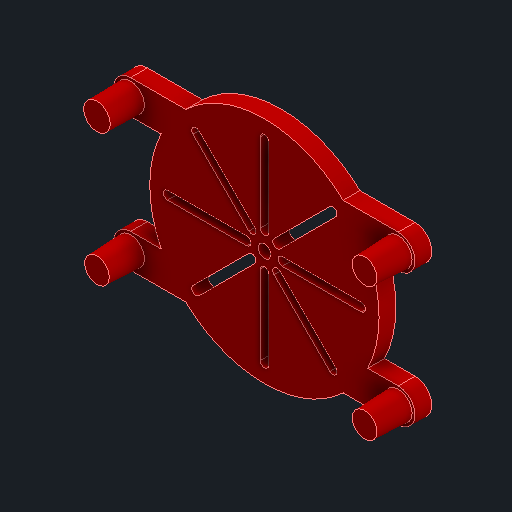
# Autodesk Inventor part: Laser Alignment Tool V2
Saved by Autodesk Inventor 2023.4 (Build 274418000, 418)
## iProperties
Created: 2022-11-15
Part Number: Laser Alignment Tool V2
Material: Generic
Document SubType Name: Modeling
Designer: xSibe
Density: 1 g/cm^3
Appearance: Plastic Dark Red
Author: xSibe
Autodesk Inventor part; units mm, degrees
ref_plane "YZ Plane" through (0, 0, 0) normal (1, 0, 0) x (0, 1, 0)
ref_plane "XZ Plane" through (0, 0, 0) normal (0, 1, 0) x (-1, 0, 0)
ref_plane "XY Plane" through (0, 0, 0) normal (0, 0, 1) x (1, 0, 0)
sketch "Sketch2" plane through (0, 0, 0) normal (0, 0, 1) x (0, 1, 0)
  line L0 (7.7, -24.9) -> (42.1, -24.9) projected
  line L1 (7.7, -24.9) -> (42.1, -24.9) projected
  circle A0 centre (34.8, 19.9) radius 2.0625 projected
  circle A1 centre (15, 19.9) radius 2.0625 projected
  circle A2 centre (15, -19.9) radius 2.0625 projected
  circle A3 centre (34.8, -19.9) radius 2.0625 projected
  line L2 (7.7, 17.05) -> (42.1, 17.05) projected
  line L3 (7.7, -17.05) -> (42.1, -17.05) projected
  line L4 (24.9, 17.05) -> (24.9, -17.05)
  circle A4 centre (24.9, 0) radius 17.05
  circle A5 centre (24.9, 0) radius 0.9375
  line L5 (24.9, 0) -> (36.9562, -12.0562)
  line L6 (24.9, 0) -> (41.95, 0) construction
  line L7 (26.7738, -1.8738) -> (35.0823, -10.1823) construction
  line L8 (26.3319, -2.3158) -> (34.6404, -10.6243)
  line L9 (35.5243, -9.7404) -> (27.2158, -1.4319)
  arc A6 (27.2158, -1.4319) -> (26.3319, -2.3158) centre (26.7738, -1.8738) ccw
  arc A7 (34.6404, -10.6243) -> (35.5243, -9.7404) centre (35.0823, -10.1823) ccw
  line L10 (30.9281, -6.0281) -> (42.6781, -6.0281) construction
  line L11 (34.8, 19.9) -> (34.8, 13.8814) construction
  line L12 (32.3, 19.9) -> (32.3, 13.8814)
  line L13 (37.3, 13.8814) -> (37.3, 19.9)
  arc A8 (37.3, 19.9) -> (32.3, 19.9) centre (34.8, 19.9) ccw
  arc A9 (32.3, 13.8814) -> (37.3, 13.8814) centre (34.8, 13.8814) ccw
  line L14 (15, 19.9) -> (15, 13.8814) construction
  line L15 (12.5, 19.9) -> (12.5, 13.8814)
  line L16 (17.5, 13.8814) -> (17.5, 19.9)
  arc A10 (17.5, 19.9) -> (12.5, 19.9) centre (15, 19.9) ccw
  arc A11 (12.5, 13.8814) -> (17.5, 13.8814) centre (15, 13.8814) ccw
  line L17 (15, -19.9) -> (15, -13.8814) construction
  line L18 (17.5, -19.9) -> (17.5, -13.8814)
  line L19 (12.5, -13.8814) -> (12.5, -19.9)
  arc A12 (12.5, -19.9) -> (17.5, -19.9) centre (15, -19.9) ccw
  arc A13 (17.5, -13.8814) -> (12.5, -13.8814) centre (15, -13.8814) ccw
  line L20 (34.8, -19.9) -> (34.8, -13.8814) construction
  line L21 (37.3, -19.9) -> (37.3, -13.8814)
  line L22 (32.3, -13.8814) -> (32.3, -19.9)
  arc A14 (32.3, -19.9) -> (37.3, -19.9) centre (34.8, -19.9) ccw
  arc A15 (37.3, -13.8814) -> (32.3, -13.8814) centre (34.8, -13.8814) ccw
  line L23 (39.3, 0.625) -> (27.55, 0.625)
  arc A16 (39.3, -0.625) -> (39.3, 0.625) centre (39.3, 0) ccw
  line L24 (27.55, -0.625) -> (39.3, -0.625)
  arc A17 (27.55, 0.625) -> (27.55, -0.625) centre (27.55, 0) ccw
  line L25 (34.6404, 10.6243) -> (26.3319, 2.3158)
  arc A18 (35.5243, 9.7404) -> (34.6404, 10.6243) centre (35.0823, 10.1823) ccw
  line L26 (27.2158, 1.4319) -> (35.5243, 9.7404)
  arc A19 (26.3319, 2.3158) -> (27.2158, 1.4319) centre (26.7738, 1.8738) ccw
  line L27 (24.275, 14.4) -> (24.275, 2.65)
  arc A20 (25.525, 14.4) -> (24.275, 14.4) centre (24.9, 14.4) ccw
  line L28 (25.525, 2.65) -> (25.525, 14.4)
  arc A21 (24.275, 2.65) -> (25.525, 2.65) centre (24.9, 2.65) ccw
  line L29 (14.2757, 9.7404) -> (22.5842, 1.4319)
  arc A22 (15.1596, 10.6243) -> (14.2757, 9.7404) centre (14.7177, 10.1823) ccw
  line L30 (23.4681, 2.3158) -> (15.1596, 10.6243)
  arc A23 (22.5842, 1.4319) -> (23.4681, 2.3158) centre (23.0262, 1.8738) ccw
  line L31 (10.5, -0.625) -> (22.25, -0.625)
  arc A24 (10.5, 0.625) -> (10.5, -0.625) centre (10.5, 0) ccw
  line L32 (22.25, 0.625) -> (10.5, 0.625)
  arc A25 (22.25, -0.625) -> (22.25, 0.625) centre (22.25, 0) ccw
  line L33 (15.1596, -10.6243) -> (23.4681, -2.3158)
  arc A26 (14.2757, -9.7404) -> (15.1596, -10.6243) centre (14.7177, -10.1823) ccw
  line L34 (22.5842, -1.4319) -> (14.2757, -9.7404)
  arc A27 (23.4681, -2.3158) -> (22.5842, -1.4319) centre (23.0262, -1.8738) ccw
  line L35 (25.525, -14.4) -> (25.525, -2.65)
  arc A28 (24.275, -14.4) -> (25.525, -14.4) centre (24.9, -14.4) ccw
  line L36 (24.275, -2.65) -> (24.275, -14.4)
  arc A29 (25.525, -2.65) -> (24.275, -2.65) centre (24.9, -2.65) ccw
  line L37 (37.3, 13.8814) -> (37.3, -13.8814)
  line L38 (12.5, -13.8814) -> (12.5, 13.8814)
  point P0 (0, 0)
  point P1 (34.8, 16.8907)
  point P2 (15, 16.8907)
  point P3 (15, -16.8907)
  point P4 (34.8, -16.8907)
  point P5 (17.5, 15.3604)
  point P6 (13.0765, 12.2844)
  point P7 (13.0765, -12.2844)
  point P8 (17.5, -15.3604)
  point P9 (32.3, -15.3604)
  point P10 (36.7235, -12.2844)
  point P11 (36.7235, 12.2844)
  point P12 (32.3, 15.3604)
  point P13 (12.5, 11.7022)
  point P14 (12.5, -11.7022)
  point P15 (37.3, -11.7022)
  point P16 (37.3, 11.7022)
  dimension "d32" = 1.875
  dimension "d33" = 45
  dimension "d34" = 5.875
  dimension "d35" = 45
  dimension "d36" = 1.25
  dimension "d37" = 5
  dimension "d38" = 5
  dimension "d39" = 5
  dimension "d40" = 5
  dimension "d43" = 360
  constraints: 80 end point, 54 point on circle, 26 centre point, 20 tangent, 9 midpoint, 6 parallel, 2 coincident, 2 equal length, 2 horizontal, 2 point on line, 1 collinear, 1 vertical, 81 other
  measures "d32" diameter of A5
  measures "d33" angle of L5 L6
  measures "d34" distance of L10.start L7.end
  measures "d35" angle of L7 L10
  measures "d36" diameter of A7
  measures "d37" diameter of A9
  measures "d38" diameter of A11
  measures "d39" diameter of A13
  measures "d40" diameter of A15
extrude "Extrusion2" add sketch "Sketch2" along normal mid plane 2.5 contours A0 | A1 | A2 | A3 | L15 A10 L16 L2 | L2 L16 A4 A11 L15 | A11 A4 L38 | A4 L12 A9 L37 L23 A17 L24 L5 A7 L9 A6 A5 L4 A21 L28 A20 | L4 A20 L27 A21 A5 A29 L36 A28 A4 L18 A13 L38 L31 A25 L32 A11 L16 | L16 A11 A4 | L38 L32 A24 L31 A4 | L12 A8 L13 L2 | L2 L13 A9 A4 L12 | A4 A9 L12 | A4 A13 L38 | A9 L37 A4 | A13 L18 A4 | A4 L18 L3 L19 A13 | A4 L37 L24 A16 L23 | L3 L18 A12 L19 | A5 L5 A6 L8 A7 A4 A15 L22 L4 A28 L35 A29 | L37 A15 A4 | L22 A4 A15 L21 L3 | L3 L21 A14 L22 | L22 A15 A4
sketch "Sketch3" plane through (0, 0, 1.25) normal (0, 0, 1) x (1, 0, 0)
  circle A0 centre (-19.9, 34.8) radius 2.0625 projected
  circle A1 centre (-19.9, 15) radius 2.0625 projected
  circle A2 centre (19.9, 15) radius 2.0625 projected
  circle A3 centre (19.9, 34.8) radius 2.0625 projected
  point P0 (0, 0)
extrude "Extrusion3" add sketch "Sketch3" along normal blind 5
chamfer "Chamfer1" distance 5 angle 1 1 edges at (-21.9625, 34.8, 6.25) measured on face at (-21.9625, 34.8, 5.75)
chamfer "Chamfer2" distance 5 angle 2.5 1 edges at (-21.9625, 15, 6.25) measured on face at (-21.9625, 15, 5.75)
chamfer "Chamfer3" distance 5 angle 2.5 1 edges at (17.8375, 15, 6.25) measured on face at (17.8375, 15, 5.75)
chamfer "Chamfer4" distance 5 angle 2.5 1 edges at (17.8375, 34.8, 6.25) measured on face at (17.8375, 34.8, 5.75)
body "Solid1"
